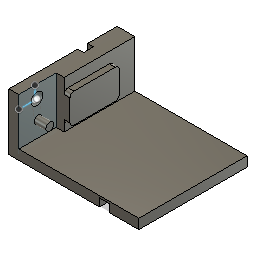
GoPro Mount Cover (Autodesk Fusion 360 design; units mm, degrees)
Autodesk Fusion 360 part; units mm, degrees
sketch "Sketch1" plane through (0, 0, 0) normal (0, 1, 0) x (1, 0, 0)
  line L0 (-40, 35) -> (31, 35)
  line L1 (31, 35) -> (31, -20)
  line L2 (31, -20) -> (-40, -20)
  line L3 (-40, -20) -> (-40, 35)
  line L4 (-40, 35) -> (-45, 35)
  line L5 (-45, 35) -> (-45, -20)
  line L6 (-45, -20) -> (-40, -20)
  line L7 (-40, -20) -> (-40, 35)
  dimension "d1" = 71
  dimension "d2" = 55
  constraint perpendicular L0 L1
  constraint parallel L0 L2
  constraint parallel L1 L3
  constraint horizontal L0
  constraint perpendicular L4 L5
  constraint parallel L4 L6
  constraint parallel L5 L7
  constraint perpendicular L3 L4
  measures "d1" distance of L0.start L0.end
  measures "d2" distance of L0.start L2.end
extrude "Extrude1" add sketch "Sketch1" along normal blind 3 contours L0 L1 L2 L3 L7 makes body 1
extrude "Extrude2" add sketch "Sketch1" along normal blind 3 contours L3 L4 L5 L6 L7 bodies 1
extrude "Extrude3" add sketch "Sketch1" along normal blind 29 separate body contours L3 L4 L5 L6 L7 makes body 2
sketch "Sketch2" plane through (-40, 0, 0) normal (1, 0, 0) x (0, 0, -1)
  line L0 (-20, 0) -> (35, 0)
  line L1 (35, 0) -> (35, 29)
  line L2 (35, 29) -> (-20, 29)
  line L3 (-20, 29) -> (-20, 0)
  line L4 (35, 29) -> (-1, 29)
  line L5 (-1, 29) -> (-1, 3)
  line L6 (-1, 3) -> (35, 3)
  line L7 (35, 3) -> (35, 29)
  line L8 (-20, 3) -> (35, 3)
  dimension "d9" = 36
  constraint perpendicular L4 L5
  constraint parallel L4 L6
  constraint parallel L5 L7
  constraint perpendicular L1 L4
  constraint coincident L1.end L2.start
  measures "d9" distance of L1.end L4.end
extrude "Extrude4" add sketch "Sketch2" along normal blind 4 contours L1 L2 L4 L5 L6 L7 L8 bodies 1 2
sketch "Sketch3" plane through (-36, 0, 0) normal (1, 0, 0) x (0, 0, -1)
  line L0 (-1, 29) -> (-1, 3)
  line L1 (-1, 3) -> (35, 3)
  line L2 (35, 3) -> (35, 29)
  line L3 (35, 29) -> (-1, 29)
  line L4 (20.1451, 29) -> (20.1451, 23.5)
  line L5 (-1, 23.5) -> (24, 23.5)
  line L6 (24, 23.5) -> (24, 8.5)
  line L7 (24, 8.5) -> (-1, 8.5)
  line L8 (-1, 8.5) -> (-1, 23.5)
  dimension "d12" = 5.5
  dimension "d13" = 25
  dimension "d14" = 15
  constraint coincident L3 L4.start
  constraint perpendicular L5 L6
  constraint parallel L5 L7
  constraint parallel L6 L8
  constraint perpendicular L0 L5
  constraint coincident L0 L5.start
  measures "d12" distance of L4.start L4.end
  measures "d13" distance of L5.start L5.end
  measures "d14" distance of L5.start L7.end
extrude "Extrude5" add sketch "Sketch3" along normal blind 3 contours L0 L5 L6 L7 L8 bodies 1
fillet "Fillet1" radius 2 4 edges at (-34.5, 23.5, 1) (-34.5, 8.5, 1) (-34.5, 23.5, -24) (-34.5, 8.5, -24) on bodies 1
sketch "Sketch4" plane through (-40, 0, 0) normal (1, 0, 0) x (0, 0, -1)
  line L0 (-20, 3) -> (-1, 3)
  line L1 (-1, 3) -> (-1, 29)
  line L2 (-1, 29) -> (-20, 29)
  line L3 (-20, 29) -> (-20, 3)
  line L4 (-11.8235, 29) -> (-11.8235, 22.5)
  line L5 (-20, 22.5122) -> (-10.75, 22.5122)
  dimension "d18" = 6.5
  dimension "d19" = 9.25
  constraint coincident L2 L4.start
  constraint coincident L3 L5.start
  measures "d18" distance of L4.start L4.end
  measures "d19" distance of L5.start L5.end
sketch "Sketch5" plane through (-45, 0, 0) normal (-1, 0, 0) x (0, 0, 1)
  line L0 (-35, 0) -> (20, 0)
  line L1 (20, 0) -> (20, 29)
  line L2 (20, 29) -> (-35, 29)
  line L3 (-35, 29) -> (-35, 0)
  line L4 (8.25, 22.5122) -> (8.25, 13.0122)
  line L5 (8.25, 13.0122) -> (10.25, 13.0122)
  dimension "d22" = 9.5
  dimension "d23" = 2
  measures "d22" distance of L4.start L4.end
  measures "d23" distance of L4.end L5.end
cylinder "CylinderPrimitive2" add diameter 4 height 6 placed x (0, 0, -1) y (0, 1, 0) z (1, 0, 0) at (-40, 13.0122, 10.25) bodies 1
extrude "Extrude6" add 1 faces at (8.6667, 3, -4.6667) along direction (0, 1, 0) blind 2 on bodies 1 bodies 1
extrude "Extrude7" cut 1 faces at (5.6667, 0, 1.6667) along direction (0, 1, 0) blind 2 on bodies 1 bodies 1
cylinder "CylinderPrimitive3" cut diameter 6 height -6 placed x (0, 0, -1) y (0, 1, 0) z (1, 0, 0) at (-40, 22.5122, 10.75) bodies 1
extrude "Extrude8" add 1 faces at (5.6667, 2, 1.6667) along direction (0, -1, 0) blind 2 on bodies 1 bodies 1
sketch "Sketch8" plane through (0, 0, 0) normal (0, -1, 0) x (1, 0, 0)
  line L0 (-45, -35) -> (31, -35)
  line L1 (31, -35) -> (31, 20)
  line L2 (31, 20) -> (-45, 20)
  line L3 (-45, 20) -> (-45, -35)
  line L4 (31, 20) -> (6, 20)
  line L5 (6, 20) -> (1, 20)
  line L6 (1, 20) -> (1, -35)
  line L7 (1, -35) -> (6, -35)
  line L8 (6, -35) -> (6, 20)
  dimension "d34" = 25
  dimension "d35" = 5
  constraint coincident L1.end L2.start
  constraint perpendicular L5 L6
  constraint parallel L5 L7
  constraint parallel L6 L8
  constraint parallel L2 L5
  measures "d34" distance of L1.end L4.end
  measures "d35" distance of L4.end L5.end
extrude "Extrude9" cut sketch "Sketch8" against normal blind 2 contours L0 L2 L5 L6 L7 L8 bodies 1
chamfer "Chamfer1" distance 2 angle 45 2 edges at (3.5, 2, 20) (3.5, 2, -35) on bodies 1
extrude "Extrude10" cut 1 faces at (31, 3.3333, -16.6667) along direction (-1, 0, 0) blind 10 on bodies 1 bodies 1
sketch "Sketch9" plane through (-45, 0, 0) normal (-1, 0, 0) x (0, 0, 1)
  circle A0 centre (10.75, 22.5122) radius 3
  line L0 (20, 0) -> (20, 29)
  line L1 (20, 29) -> (-35, 29)
  line L2 (-35, 29) -> (-35, 0)
  line L3 (-35, 0) -> (20, 0)
  line L4 (-20, 29) -> (-15, 29)
  line L5 (-15, 29) -> (-20, 29)
  line L6 (-20, 29) -> (-20, 0)
  line L7 (-20, 0) -> (-15, 0)
  line L8 (-15, 0) -> (-15, 29)
  dimension "d41" = 20
  constraint perpendicular L5 L6
  constraint parallel L5 L7
  constraint parallel L6 L8
  measures "d41" distance of L1.end L4.end
extrude "Extrude11" cut sketch "Sketch9" against normal blind 1 contours L1 L3 L4 L5 L6 L7 L8 bodies 1
chamfer "Chamfer2" distance 2 angle 45 2 edges at (-44, 29, -17.5) (-44, 0, -17.5) on bodies 1
